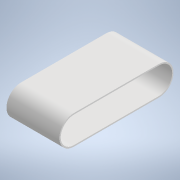
# Autodesk Inventor part: Förderband
Saved by Autodesk Inventor 2021 (Build 250183000, 183)
## iProperties
Created: 2022-06-27
Part Number: Förderband
Material: Generisch
Document SubType Name: Modeling
Designer: adria
Mass: 7778.47 g
Surface Area: 15945.9 cm^2
Volume: 7778.47 cm^3
Density: 1 g/cm^3
Appearance: Vorgabe
Author: adria
Autodesk Inventor part; units mm, degrees
ref_plane "YZ Plane" through (0, 0, 0) normal (1, 0, 0) x (0, 1, 0)
ref_plane "XZ Plane" through (0, 0, 0) normal (0, 1, 0) x (-1, 0, 0)
ref_plane "XY Plane" through (0, 0, 0) normal (0, 0, 1) x (1, 0, 0)
sketch "Skizze3" plane through (0, 0, 0) normal (1, 0, 0) x (0, 1, 0)
  line L0 (-97.3116, 946.0308) -> (-97.3116, 624.8101)
  arc A0 (-297.3116, 624.8101) -> (-97.3116, 624.8101) centre (-197.3116, 624.8101) ccw
  line L1 (-297.3116, 624.8101) -> (-297.3116, 1009.2763)
  line L2 (-97.3116, 946.0308) -> (-97.3116, 1267.2514)
  arc A1 (-97.3116, 1267.2514) -> (-297.3116, 1267.2514) centre (-197.3116, 1267.2514) ccw
  line L3 (-297.3116, 1267.2514) -> (-297.3116, 1009.2763)
  line L4 (-87.3116, 946.0308) -> (-87.3116, 624.8101)
  arc A2 (-307.3116, 624.8101) -> (-87.3116, 624.8101) centre (-197.3116, 624.8101) ccw
  line L5 (-307.3116, 624.8101) -> (-307.3116, 946.0308)
  line L6 (-87.3116, 946.0308) -> (-307.3116, 946.0308)
  line L7 (-307.3116, 1267.2514) -> (-307.3116, 946.0308)
  line L8 (-87.3116, 946.0308) -> (-87.3116, 1267.2514)
  arc A3 (-87.3116, 1267.2514) -> (-307.3116, 1267.2514) centre (-197.3116, 1267.2514) ccw
  point P0 (0, 0)
  dimension "d0" = 110
  dimension "d1" = 100
  constraints: 18 end point, 8 point on circle, 6 tangent, 4 centre point, 3 symmetric about line, 2 coincident, 2 vertical, 1 horizontal, 1 other
  measures "d0" radius of A2
  measures "d1" radius of A0
extrude "Extrusion1" add sketch "Skizze3" along normal mid plane 400 contours L6 L4 A2 L5 L1 A0 L0 | L2 A1 L3 L1 L6 L7 A3 L8
